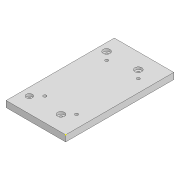
# Autodesk Inventor part: suporte-fonte2
Saved by Autodesk Inventor 2020 (Build 240168000, 168)
## iProperties
Created: 2022-07-23
Part Number: suporte-fonte2
Material: Genérico
Document SubType Name: Modeling
Designer: gabri
Density: 1 g/cm^3
Appearance: Padrão
Author: gabri
Autodesk Inventor part; units mm, degrees
ref_plane "YZ Plane" through (0, 0, 0) normal (1, 0, 0) x (0, 1, 0)
ref_plane "XZ Plane" through (0, 0, 0) normal (0, 1, 0) x (-1, 0, 0)
ref_plane "XY Plane" through (0, 0, 0) normal (0, 0, 1) x (1, 0, 0)
sketch "Esboço1" plane through (0, 0, 0) normal (0, 1, 0) x (-1, 0, 0)
  line L0 (0, 0) -> (77, 0)
  line L1 (77, 0) -> (77, -140)
  line L2 (77, -140) -> (0, -140)
  line L3 (0, -140) -> (0, 0)
  circle A0 centre (67, -20) radius 2
  circle A1 centre (67, -120) radius 2
  circle A2 centre (26, -20) radius 2
  circle A3 centre (26, -120) radius 2
  dimension "d0" = 77
  dimension "d1" = 140
  dimension "d2" = 4
  dimension "d3" = 4
  dimension "d4" = 4
  dimension "d5" = 4
  dimension "d6" = 10
  dimension "d7" = 10
  dimension "d8" = 20
  dimension "d9" = 20
  dimension "d10" = 20
  dimension "d11" = 20
  dimension "d12" = 26
  dimension "d13" = 26
  constraints: 8 end point, 4 centre point, 2 parallel, 1 horizontal, 1 perpendicular
  measures "d0" distance of L0.start L0.end
  measures "d1" distance of L0.end L1.end
  measures "d2" diameter of A0
  measures "d3" diameter of A1
  measures "d4" diameter of A2
  measures "d5" diameter of A3
  measures "d6" distance from line of L1 A0.centre
  measures "d7" distance from line of L1 A1.centre
  measures "d8" distance from line of L2 A1.centre
  measures "d9" distance from line of L0 A0.centre
  measures "d10" distance from line of L0 A2.centre
  measures "d11" distance from line of L2 A3.centre
  measures "d12" distance from line of L3 A2.centre
  measures "d13" distance from line of L3 A3.centre
extrude "Extrusão1" add sketch "Esboço1" along normal blind 8
sketch "Esboço2" plane through (0, 8, 0) normal (0, 1, 0) x (1, 0, 0)
  circle A0 centre (-67, 20) radius 2 projected
  circle A1 centre (-26, 20) radius 2 projected
  circle A2 centre (-26, 120) radius 2 projected
  circle A3 centre (-67, 120) radius 2 projected
  circle A4 centre (-67, 20) radius 4
  circle A5 centre (-67, 120) radius 2 projected
  circle A6 centre (-67, 120) radius 4.5
  circle A7 centre (-26, 120) radius 2 projected
  circle A8 centre (-26, 120) radius 4.5
  circle A9 centre (-26, 20) radius 2 projected
  circle A10 centre (-26, 20) radius 4.5
  point P0 (0, 0)
  dimension "d16" = 8
  dimension "d17" = 9
  dimension "d18" = 9
  dimension "d19" = 9
  constraints: 4 centre point, 4 coincident
  measures "d16" diameter of A4
  measures "d17" diameter of A6
  measures "d18" diameter of A8
  measures "d19" diameter of A10
extrude "Extrusão2" cut sketch "Esboço2" against normal blind 3 contours A3 | A4 | A6 | A8 | A10
sketch "Esboço3" plane through (0, 8, 0) normal (0, 1, 0) x (1, 0, 0)
  point P0 (0, 0)
sketch "Esboço4" plane through (0, 8, 0) normal (0, 1, 0) x (1, 0, 0)
  circle A0 centre (-57, 30) radius 2
  circle A1 centre (-57, 110) radius 2
  circle A2 centre (-67, 20) radius 2 projected
  circle A3 centre (-67, 120) radius 2 projected
  circle A4 centre (-16, 30) radius 2
  circle A5 centre (-16, 110) radius 2
  circle A6 centre (-26, 20) radius 2 projected
  circle A7 centre (-26, 120) radius 2 projected
  point P0 (0, 0)
  dimension "d22" = 4
  dimension "d23" = 4
  dimension "d24" = 10
  dimension "d25" = 10
  dimension "d26" = 10
  dimension "d27" = 10
  dimension "d28" = 4
  dimension "d29" = 4
  dimension "d30" = 10
  dimension "d31" = 10
  dimension "d32" = 10
  dimension "d33" = 10
  constraints: 4 centre point
  measures "d22" diameter of A0
  measures "d23" diameter of A1
  measures "d24" horizontal distance of A0.centre A2.centre
  measures "d25" horizontal distance of A0.centre A2.centre
  measures "d26" horizontal distance of A3.centre A1.centre
  measures "d27" horizontal distance of A3.centre A1.centre
  measures "d28" diameter of A4
  measures "d29" diameter of A5
  measures "d30" horizontal distance of A4.centre A6.centre
  measures "d31" horizontal distance of A4.centre A6.centre
  measures "d32" horizontal distance of A7.centre A5.centre
  measures "d33" horizontal distance of A7.centre A5.centre
extrude "Extrusão3" cut sketch "Esboço4" against normal blind 12 contours A0 | A1 | A4 | A5
sketch "Esboço5" plane through (0, 0, 0) normal (0, -1, 0) x (1, 0, 0)
  circle A0 centre (-57, -110) radius 2 projected
  circle A1 centre (-16, -110) radius 2 projected
  circle A2 centre (-16, -30) radius 2 projected
  circle A3 centre (-57, -30) radius 2 projected
  line L0 (-53.525, -112.0063) -> (-57, -114.0126)
  line L1 (-57, -114.0126) -> (-60.475, -112.0063)
  line L2 (-60.475, -112.0063) -> (-60.475, -107.9937)
  line L3 (-60.475, -107.9937) -> (-57, -105.9874)
  line L4 (-57, -105.9874) -> (-53.525, -107.9937)
  line L5 (-53.525, -107.9937) -> (-53.525, -112.0063)
  line L6 (-53.525, -32.0063) -> (-57, -34.0126)
  line L7 (-57, -34.0126) -> (-60.475, -32.0063)
  line L8 (-60.475, -32.0063) -> (-60.475, -27.9937)
  line L9 (-60.475, -27.9937) -> (-57, -25.9874)
  line L10 (-57, -25.9874) -> (-53.525, -27.9937)
  line L11 (-53.525, -27.9937) -> (-53.525, -32.0063)
  line L12 (-16, -105.9874) -> (-12.525, -107.9937)
  line L13 (-12.525, -107.9937) -> (-12.525, -112.0063)
  line L14 (-12.525, -112.0063) -> (-16, -114.0126)
  line L15 (-16, -114.0126) -> (-19.475, -112.0063)
  line L16 (-19.475, -112.0063) -> (-19.475, -107.9937)
  line L17 (-19.475, -107.9937) -> (-16, -105.9874)
  circle A4 centre (-16, -30) radius 2 projected
  line L18 (-12.525, -32.0063) -> (-16, -34.0126)
  line L19 (-16, -34.0126) -> (-19.475, -32.0063)
  line L20 (-19.475, -32.0063) -> (-19.475, -27.9937)
  line L21 (-19.475, -27.9937) -> (-16, -25.9874)
  line L22 (-16, -25.9874) -> (-12.525, -27.9937)
  line L23 (-12.525, -27.9937) -> (-12.525, -32.0063)
  line L24 (-77, -140) -> (-77, 0) projected
  line L25 (0, 0) -> (0, -140) projected
  dimension "d36" = 6.95
  dimension "d37" = 6.95
  dimension "d38" = 6.95
  dimension "d39" = 6.95
  constraints: 48 end point, 4 coincident, 4 parallel, 52 other
  measures "d36" distance between parallel lines of L5 L2
  measures "d37" distance between parallel lines of L11 L8
  measures "d38" distance between parallel lines of L13 L16
  measures "d39" distance between parallel lines of L22 L19
extrude "Extrusão4" cut sketch "Esboço5" against normal blind 5 contours A0 | L0 L1 L2 L3 L4 L5 | L6 L7 L8 L9 L10 L11 | L12 L13 L14 L15 L16 L17 | L18 L19 L20 L21 L22 L23
equation "\"d4\" = d3"
equation "\"d5\" = d3"
equation "\"d7\" = d6"
equation "\"d9\" = d8"
equation "\"d10\" = d9"
equation "\"d11\" = d8"
equation "\"d26\" = d25"
equation "\"d27\" = d26"
equation "\"d30\" = d24"
equation "\"d33\" = d32"
equation "\"d36\" = d39"
equation "\"d37\" = d39"
equation "\"d38\" = d39"
